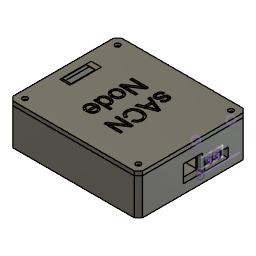
sACN Node 3xXLR_v31 (Autodesk Fusion 360 design; units mm, degrees)
Autodesk Fusion 360 part; units mm, degrees
(part 1 of 2)
sketch "Skizze1" plane through (0, 0, 0) normal (0, 1, 0) x (1, 0, 0) in component "Board"
  line L0 (99.5, 0) -> (99.5, 67)
  line L1 (99.5, 67) -> (99.5, 42.25) construction
  line L2 (99.5, 42.25) -> (99.5, 25.5) construction
  line L3 (99.5, 25.5) -> (99.5, 0) construction
  line L4 (99.5, 42.25) -> (101, 42.25)
  line L5 (101, 42.25) -> (101, 26.25)
  line L6 (101, 26.25) -> (99.5, 26.25)
  line L7 (99.5, 26.25) -> (99.5, 42.25) construction
  line L8 (99.5, 67) -> (99.5, 60.5) construction
  line L9 (99.5, 47.25) -> (99.5, 60.5)
  line L10 (99.5, -28.5) -> (0, -28.5)
  line L11 (0, 95.5) -> (99.5, 95.5)
  line L12 (99.5, 95.5) -> (99.5, -28.5)
  line L13 (0, 95.5) -> (-50, 95.5)
  line L14 (-50, 95.5) -> (-50, -28.5)
  line L15 (-50, -28.5) -> (0, -28.5)
  line L16 (0, 100.5) -> (104.5, 100.5)
  line L17 (104.5, 100.5) -> (104.5, -33.5)
  line L18 (104.5, -33.5) -> (0, -33.5)
  line L19 (-55, -33.5) -> (0, -33.5)
  line L20 (-55, 100.5) -> (-55, -33.5)
  line L21 (0, 100.5) -> (-55, 100.5)
  line L22 (99.5, 62) -> (99.5, 67)
  line L23 (99.5, 5) -> (99.5, 0)
  line L24 (99.5, 0) -> (99.5, -0.4)
  line L25 (99.5, -0.4) -> (99.5, -2.4)
  line L26 (99.5, 67.4) -> (99.5, 69.4)
  line L27 (99.5, 67) -> (99.5, 67.4)
  line L28 (99.5, 33.5) -> (99.5, 47.25)
  line L29 (99.5, 47.25) -> (41, 47.25)
  line L30 (41, 47.25) -> (41, 21.25)
  line L31 (41, 21.25) -> (99.5, 21.25)
  line L32 (99.5, 21.25) -> (99.5, 47.25)
  circle A0 centre (97.5, 45.25) radius 1
  circle A1 centre (97.5, 23.25) radius 1
  line L33 (5.6871, 39.4777, 4.3933) -> (5.6871, 41.4777, 4.3933)
  line L34 (5.6871, 39.4777, 4.3947) -> (5.6871, 41.4777, 4.3947)
  line L35 (-22.2425, 41.4777, 4.3947) -> (-22.2425, 45.4777, 4.3947) construction
  line L36 (-6.3129, 41.4777, 4.3947) -> (-6.3129, 39.4777, 4.3947)
  line L37 (-0.3129, 46.5108, 4.3947) -> (-0.3129, 40.4777, 4.3947) construction
  line L38 (-21.0987, 63.9777, 4.3931) -> (-21.0987, 41.4777, 4.3931) construction
  line L39 (-0.3129, 46.5108, 4.3932) -> (-0.3129, 40.4777, 4.3933) construction
  line L40 (-18.5761, 41.4777, 4.3947) -> (-18.5761, 33.4777, 4.3947) construction
  line L41 (5.6871, 45.5113, 4.3947) -> (5.6871, 47.5113, 4.3947)
  line L42 (16.2858, 41.4777, 4.3931) -> (16.2858, 63.9777, 4.3931) construction
  line L43 (-11.4093, 33.4777, 4.3934) -> (-11.4093, 41.4777, 4.3932) construction
  line L44 (5.6871, 45.5103, 4.3934) -> (5.6871, 47.5122, 4.393)
  line L45 (-6.3129, 47.5113, 4.3947) -> (-6.3129, 45.5113, 4.3947)
  line L46 (-6.3129, 41.4777, 4.3933) -> (-6.3129, 39.4777, 4.3933)
  line L47 (-18.5761, 33.4777, 4.3934) -> (-11.4093, 33.4777, 4.3934) construction
  line L48 (-6.3129, 47.5122, 4.393) -> (5.6871, 45.5103, 4.3934) construction
  line L49 (5.6871, 41.4777, 4.3933) -> (-6.3129, 41.4777, 4.3933)
  line L50 (5.6871, 47.5122, 4.393) -> (-6.3129, 45.5103, 4.3934) construction
  line L51 (21.2575, 45.4777, 4.3934) -> (-22.2425, 41.4777, 4.3931) construction
  line L52 (-18.5761, 41.4777, 4.3932) -> (-18.5761, 33.4777, 4.3934) construction
  line L53 (-6.3129, 39.4777, 4.3933) -> (5.6871, 39.4777, 4.3933)
  line L54 (-21.0987, 41.4777, 4.3931) -> (16.2858, 41.4777, 4.3931) construction
  line L55 (5.6871, 47.5113, 4.3947) -> (-6.3129, 47.5113, 4.3947)
  line L56 (-18.5761, 33.4777, 4.3947) -> (-11.4093, 33.4777, 4.3947) construction
  line L57 (-11.4093, 33.4777, 4.3947) -> (-11.4093, 41.4777, 4.3947) construction
  line L58 (-22.2425, 45.4777, 4.3947) -> (21.2575, 45.4777, 4.3947) construction
  line L59 (21.2575, 45.4777, 4.3947) -> (-22.2425, 41.4777, 4.3947) construction
  line L60 (-6.3129, 47.5122, 4.393) -> (-6.3129, 45.5103, 4.3934)
  line L61 (-6.3129, 47.5113, 4.3947) -> (5.6871, 45.5113, 4.3947) construction
  line L62 (-22.2425, 41.4777, 4.3931) -> (-22.2425, 45.4777, 4.3931) construction
  line L63 (21.2575, 45.4777, 4.3947) -> (21.2575, 41.4777, 4.3947) construction
  line L64 (21.2575, 45.4777, 4.3934) -> (21.2575, 41.4777, 4.3934) construction
  line L65 (5.6871, 47.5113, 4.3947) -> (-6.3129, 45.5113, 4.3947) construction
  line L66 (-22.2425, 45.4777, 4.3931) -> (21.2575, 41.4777, 4.3934) construction
  line L67 (-6.3129, 45.5113, 4.3947) -> (5.6871, 45.5113, 4.3947)
  line L68 (21.2575, 41.4777, 4.3947) -> (-22.2425, 41.4777, 4.3947) construction
  line L69 (-6.3129, 41.4777, 4.3933) -> (5.6871, 39.4777, 4.3933) construction
  line L70 (16.2858, 63.9777, 4.3931) -> (-21.0987, 63.9777, 4.3931) construction
  line L71 (5.6871, 47.5122, 4.393) -> (-6.3129, 47.5122, 4.393)
  line L72 (5.6871, 41.4777, 4.3947) -> (-6.3129, 41.4777, 4.3947)
  line L73 (-22.2425, 45.4777, 4.3947) -> (21.2575, 41.4777, 4.3947) construction
  line L74 (-6.3129, 45.5103, 4.3934) -> (5.6871, 45.5103, 4.3934)
  line L75 (-6.3129, 41.4777, 4.3947) -> (5.6871, 39.4777, 4.3947) construction
  line L76 (21.2575, 41.4777, 4.3934) -> (-22.2425, 41.4777, 4.3931) construction
  line L77 (-22.2425, 45.4777, 4.3931) -> (21.2575, 45.4777, 4.3934) construction
  line L78 (-6.3129, 39.4777, 4.3947) -> (5.6871, 39.4777, 4.3947)
  line L79 (5.6871, 41.4777, 4.3933) -> (-6.3129, 39.4777, 4.3933) construction
  line L80 (5.6871, 41.4777, 4.3947) -> (-6.3129, 39.4777, 4.3947) construction
  line L81 (-6.3129, 47.5113, 4.3932) -> (-6.3129, 45.5113, 4.3932)
  line L82 (5.6871, 39.4777, 4.3933) -> (5.6871, 41.4777, 4.3933)
  line L83 (5.6871, 41.4777, 4.3947) -> (-6.3129, 39.4777, 4.3947) construction
  line L84 (-22.2425, 45.4777, 4.3931) -> (21.2575, 45.4777, 4.3934) construction
  line L85 (-22.2425, 45.4777, 4.3947) -> (21.2575, 41.4777, 4.3947) construction
  line L86 (-18.5761, 41.4777, 4.3947) -> (-18.5761, 33.4777, 4.3947) construction
  line L87 (-22.2425, 45.4777, 4.3947) -> (21.2575, 45.4777, 4.3947) construction
  line L88 (5.6871, 47.5113, 4.3947) -> (-6.3129, 47.5113, 4.3947)
  line L89 (5.6871, 45.5113, 4.3932) -> (5.6871, 47.5113, 4.3932)
  line L90 (-6.3129, 41.4777, 4.3933) -> (5.6871, 39.4777, 4.3933) construction
  line L91 (5.6871, 45.5113, 4.3947) -> (5.6871, 47.5113, 4.3947)
  line L92 (-6.3129, 47.5113, 4.3947) -> (5.6871, 45.5113, 4.3947) construction
  line L93 (-6.3129, 41.4777, 4.3947) -> (5.6871, 39.4777, 4.3947) construction
  line L94 (5.6871, 41.4777, 4.3933) -> (-6.3129, 41.4777, 4.3933)
  line L95 (21.2575, 45.4777, 4.3934) -> (21.2575, 41.4777, 4.3934) construction
  line L96 (-0.3129, 46.5108, 4.3947) -> (-0.3129, 40.4777, 4.3947) construction
  line L97 (5.6871, 41.4777, 4.3933) -> (-6.3129, 39.4777, 4.3933) construction
  line L98 (-6.3129, 41.4777, 4.3933) -> (-6.3129, 39.4777, 4.3933)
  line L99 (5.6871, 41.4777, 4.3947) -> (-6.3129, 41.4777, 4.3947)
  line L100 (-6.3129, 39.4777, 4.3933) -> (5.6871, 39.4777, 4.3933)
  line L101 (5.6871, 47.5113, 4.3932) -> (-6.3129, 45.5113, 4.3932) construction
  line L102 (-6.3129, 45.5113, 4.3932) -> (5.6871, 45.5113, 4.3932)
  line L103 (-6.3129, 39.4777, 4.3947) -> (5.6871, 39.4777, 4.3947)
  line L104 (21.2575, 45.4777, 4.3947) -> (21.2575, 41.4777, 4.3947) construction
  line L105 (-6.3129, 47.5113, 4.3947) -> (-6.3129, 45.5113, 4.3947)
  line L106 (16.2858, 63.9777, 4.3931) -> (-21.0987, 63.9777, 4.3931) construction
  line L107 (-22.2425, 41.4777, 4.3947) -> (-22.2425, 45.4777, 4.3947) construction
  line L108 (21.2575, 41.4777, 4.3947) -> (-22.2425, 41.4777, 4.3947) construction
  line L109 (21.2575, 41.4777, 4.3934) -> (-22.2425, 41.4777, 4.3931) construction
  line L110 (-21.0987, 63.9777, 4.3931) -> (-21.0987, 41.4777, 4.3931) construction
  line L111 (-21.0987, 41.4777, 4.3931) -> (16.2858, 41.4777, 4.3931) construction
  line L112 (16.2858, 41.4777, 4.3931) -> (16.2858, 63.9777, 4.3931) construction
  line L113 (21.2575, 45.4777, 4.3947) -> (-22.2425, 41.4777, 4.3947) construction
  line L114 (-18.5761, 33.4777, 4.3947) -> (-11.4093, 33.4777, 4.3947) construction
  line L115 (-22.2425, 45.4777, 4.3931) -> (21.2575, 41.4777, 4.3934) construction
  line L116 (-18.5761, 41.4777, 4.3932) -> (-18.5761, 33.4777, 4.3934) construction
  line L117 (21.2575, 45.4777, 4.3934) -> (-22.2425, 41.4777, 4.3931) construction
  line L118 (-18.5761, 33.4777, 4.3934) -> (-11.4093, 33.4777, 4.3934) construction
  line L119 (-22.2425, 41.4777, 4.3931) -> (-22.2425, 45.4777, 4.3931) construction
  line L120 (5.6871, 39.4777, 4.3947) -> (5.6871, 41.4777, 4.3947)
  line L121 (-11.4093, 33.4777, 4.3934) -> (-11.4093, 41.4777, 4.3932) construction
  line L122 (5.6871, 47.5113, 4.3932) -> (-6.3129, 47.5113, 4.3932)
  line L123 (-11.4093, 33.4777, 4.3947) -> (-11.4093, 41.4777, 4.3947) construction
  line L124 (-6.3129, 47.5113, 4.3932) -> (5.6871, 45.5113, 4.3932) construction
  line L125 (-6.3129, 41.4777, 4.3947) -> (-6.3129, 39.4777, 4.3947)
  line L126 (-6.3129, 45.5113, 4.3947) -> (5.6871, 45.5113, 4.3947)
  line L127 (5.6871, 47.5113, 4.3947) -> (-6.3129, 45.5113, 4.3947) construction
  line L128 (-0.3129, 46.5108, 4.3932) -> (-0.3129, 40.4777, 4.3933) construction
  line L129 (21.2575, 14.9777, 4.3947) -> (21.2575, 10.9777, 4.3947) construction
  line L130 (-0.3129, 16.0108, 4.3947) -> (-0.3129, 9.9777, 4.3947) construction
  line L131 (-18.5761, 2.9777, 4.3934) -> (-11.4093, 2.9777, 4.3934) construction
  line L132 (-22.2425, 10.9777, 4.3931) -> (-22.2425, 14.9777, 4.3931) construction
  line L133 (-22.2425, 10.9777, 4.3931) -> (-22.2425, 14.9777, 4.3931) construction
  line L134 (21.2575, 14.9777, 4.3947) -> (21.2575, 10.9777, 4.3947) construction
  line L135 (-11.4093, 2.9777, 4.3947) -> (-11.4093, 10.9777, 4.3947) construction
  line L136 (-22.2425, 10.9777, 4.3947) -> (-22.2425, 14.9777, 4.3947) construction
  line L137 (21.2575, 14.9777, 4.3934) -> (21.2575, 10.9777, 4.3934) construction
  line L138 (-0.3129, 16.0108, 4.3932) -> (-0.3129, 9.9777, 4.3933) construction
  line L139 (-0.3129, 16.0108, 4.3947) -> (-0.3129, 9.9777, 4.3947) construction
  line L140 (21.2575, 14.9777, 4.3934) -> (21.2575, 10.9777, 4.3934) construction
  line L141 (-18.5761, 10.9777, 4.3932) -> (-18.5761, 2.9777, 4.3934) construction
  line L142 (21.2575, 14.9777, 4.3934) -> (-22.2425, 10.9777, 4.3931) construction
  line L143 (-22.2425, 14.9777, 4.3931) -> (21.2575, 14.9777, 4.3934) construction
  line L144 (21.2575, 10.9777, 4.3934) -> (-22.2425, 10.9777, 4.3931) construction
  line L145 (-22.2425, 14.9777, 4.3931) -> (21.2575, 10.9777, 4.3934) construction
  line L146 (21.2575, 14.9777, 4.3934) -> (-22.2425, 10.9777, 4.3931) construction
  line L147 (-0.3129, 16.0108, 4.3932) -> (-0.3129, 9.9777, 4.3933) construction
  line L148 (-18.5761, 2.9777, 4.3947) -> (-11.4093, 2.9777, 4.3947) construction
  line L149 (-11.4093, 2.9777, 4.3947) -> (-11.4093, 10.9777, 4.3947) construction
  line L150 (-11.4093, 2.9777, 4.3934) -> (-11.4093, 10.9777, 4.3932) construction
  line L151 (-11.4093, 2.9777, 4.3934) -> (-11.4093, 10.9777, 4.3932) construction
  line L152 (-22.2425, 10.9777, 4.3947) -> (-22.2425, 14.9777, 4.3947) construction
  line L153 (-6.3129, 17.0113, 4.3947) -> (-6.3129, 15.0113, 4.3947)
  line L154 (-6.3129, 10.9777, 4.3933) -> (5.6871, 8.9777, 4.3933) construction
  line L155 (-18.5761, 2.9777, 4.3947) -> (-11.4093, 2.9777, 4.3947) construction
  line L156 (5.6871, 15.0113, 4.3947) -> (5.6871, 17.0113, 4.3947)
  line L157 (5.6871, 17.0113, 4.3947) -> (-6.3129, 17.0113, 4.3947)
  line L158 (-18.5761, 10.9777, 4.3947) -> (-18.5761, 2.9777, 4.3947) construction
  line L159 (5.6871, 17.0113, 4.3932) -> (-6.3129, 15.0113, 4.3932) construction
  line L160 (5.6871, 10.9777, 4.3947) -> (-6.3129, 8.9777, 4.3947) construction
  line L161 (-18.5761, 2.9777, 4.3934) -> (-11.4093, 2.9777, 4.3934) construction
  line L162 (-6.3129, 15.0113, 4.3932) -> (5.6871, 15.0113, 4.3932)
  line L163 (-6.3129, 10.9777, 4.3933) -> (5.6871, 8.9777, 4.3933) construction
  line L164 (5.6871, 17.0113, 4.3932) -> (-6.3129, 15.0113, 4.3932) construction
  line L165 (-6.3129, 8.9777, 4.3933) -> (5.6871, 8.9777, 4.3933)
  line L166 (5.6871, 8.9777, 4.3947) -> (5.6871, 10.9777, 4.3947)
  line L167 (5.6871, 17.0113, 4.3932) -> (-6.3129, 17.0113, 4.3932)
  line L168 (-6.3129, 10.9777, 4.3947) -> (5.6871, 8.9777, 4.3947) construction
  line L169 (5.6871, 15.0113, 4.3932) -> (5.6871, 17.0113, 4.3932)
  line L170 (-18.5761, 10.9777, 4.3932) -> (-18.5761, 2.9777, 4.3934) construction
  line L171 (-6.3129, 15.0113, 4.3947) -> (5.6871, 15.0113, 4.3947)
  line L172 (5.6871, 10.9777, 4.3933) -> (-6.3129, 8.9777, 4.3933) construction
  line L173 (5.6871, 8.9777, 4.3933) -> (5.6871, 10.9777, 4.3933)
  line L174 (-6.3129, 17.0113, 4.3947) -> (5.6871, 15.0113, 4.3947) construction
  line L175 (-6.3129, 10.9777, 4.3947) -> (-6.3129, 8.9777, 4.3947)
  line L176 (5.6871, 17.0113, 4.3947) -> (-6.3129, 15.0113, 4.3947) construction
  line L177 (-6.3129, 17.0113, 4.3932) -> (-6.3129, 15.0113, 4.3932)
  line L178 (-6.3129, 17.0113, 4.3932) -> (5.6871, 15.0113, 4.3932) construction
  line L179 (5.6871, 8.9777, 4.3933) -> (5.6871, 10.9777, 4.3933)
  line L180 (5.6871, 8.9777, 4.3947) -> (5.6871, 10.9777, 4.3947)
  line L181 (5.6871, 10.9777, 4.3947) -> (-6.3129, 10.9777, 4.3947)
  line L182 (5.6871, 15.0113, 4.3947) -> (5.6871, 17.0113, 4.3947)
  line L183 (-6.3129, 10.9777, 4.3947) -> (5.6871, 8.9777, 4.3947) construction
  line L184 (5.6871, 15.0113, 4.3932) -> (5.6871, 17.0113, 4.3932)
  line L185 (-6.3129, 17.0113, 4.3947) -> (-6.3129, 15.0113, 4.3947)
  line L186 (5.6871, 17.0113, 4.3932) -> (-6.3129, 17.0113, 4.3932)
  line L187 (-6.3129, 8.9777, 4.3947) -> (5.6871, 8.9777, 4.3947)
  line L188 (5.6871, 17.0113, 4.3947) -> (-6.3129, 15.0113, 4.3947) construction
  line L189 (-6.3129, 17.0113, 4.3947) -> (5.6871, 15.0113, 4.3947) construction
  line L190 (-6.3129, 17.0113, 4.3932) -> (-6.3129, 15.0113, 4.3932)
  line L191 (-6.3129, 15.0113, 4.3932) -> (5.6871, 15.0113, 4.3932)
  line L192 (-6.3129, 17.0113, 4.3932) -> (5.6871, 15.0113, 4.3932) construction
  line L193 (-6.3129, 15.0113, 4.3947) -> (5.6871, 15.0113, 4.3947)
  line L194 (5.6871, 10.9777, 4.3933) -> (-6.3129, 10.9777, 4.3933)
  line L195 (5.6871, 10.9777, 4.3947) -> (-6.3129, 10.9777, 4.3947)
  line L196 (-6.3129, 10.9777, 4.3933) -> (-6.3129, 8.9777, 4.3933)
  line L197 (5.6871, 17.0113, 4.3947) -> (-6.3129, 17.0113, 4.3947)
  line L198 (-6.3129, 8.9777, 4.3947) -> (5.6871, 8.9777, 4.3947)
  line L199 (-6.3129, 10.9777, 4.3947) -> (-6.3129, 8.9777, 4.3947)
  line L200 (5.6871, 10.9777, 4.3933) -> (-6.3129, 10.9777, 4.3933)
  line L201 (-6.3129, 10.9777, 4.3933) -> (-6.3129, 8.9777, 4.3933)
  line L202 (5.6871, 10.9777, 4.3933) -> (-6.3129, 8.9777, 4.3933) construction
  line L203 (5.6871, 10.9777, 4.3947) -> (-6.3129, 8.9777, 4.3947) construction
  line L204 (-6.3129, 8.9777, 4.3933) -> (5.6871, 8.9777, 4.3933)
  line L205 (-22.2425, 14.9777, 4.3947) -> (21.2575, 14.9777, 4.3947) construction
  line L206 (21.2575, 14.9777, 4.3947) -> (-22.2425, 10.9777, 4.3947) construction
  line L207 (-22.2425, 14.9777, 4.3947) -> (21.2575, 10.9777, 4.3947) construction
  line L208 (-18.5761, 10.9777, 4.3947) -> (-18.5761, 2.9777, 4.3947) construction
  line L209 (21.2575, 10.9777, 4.3947) -> (-22.2425, 10.9777, 4.3947) construction
  line L210 (-21.0987, 10.9777, 4.3931) -> (16.2858, 10.9777, 4.3931) construction
  line L211 (21.2575, 10.9777, 4.3934) -> (-22.2425, 10.9777, 4.3931) construction
  line L212 (-21.0987, 10.9777, 4.3931) -> (16.2858, 10.9777, 4.3931) construction
  line L213 (-22.2425, 14.9777, 4.3931) -> (21.2575, 10.9777, 4.3934) construction
  line L214 (-22.2425, 14.9777, 4.3931) -> (21.2575, 14.9777, 4.3934) construction
  line L215 (16.2858, 10.9777, 4.3931) -> (16.2858, 33.4777, 4.3931) construction
  line L216 (-21.0987, 33.4777, 4.3931) -> (-21.0987, 10.9777, 4.3931) construction
  line L217 (21.2575, 14.9777, 4.3947) -> (-22.2425, 10.9777, 4.3947) construction
  line L218 (-21.0987, 33.4777, 4.3931) -> (-21.0987, 10.9777, 4.3931) construction
  line L219 (16.2858, 33.4777, 4.3931) -> (-21.0987, 33.4777, 4.3931) construction
  line L220 (16.2858, 33.4777, 4.3931) -> (-21.0987, 33.4777, 4.3931) construction
  line L221 (-22.2425, 14.9777, 4.3947) -> (21.2575, 14.9777, 4.3947) construction
  line L222 (21.2575, 10.9777, 4.3947) -> (-22.2425, 10.9777, 4.3947) construction
  line L223 (-22.2425, 14.9777, 4.3947) -> (21.2575, 10.9777, 4.3947) construction
  line L224 (16.2858, 10.9777, 4.3931) -> (16.2858, 33.4777, 4.3931) construction
  line L225 (21.2575, 75.9777, 4.3946) -> (21.2575, 71.9777, 4.3946) construction
  line L226 (-0.3132, 77.0107, 4.3946) -> (-0.3132, 70.9777, 4.3946) construction
  line L227 (-18.5761, 63.9777, 4.3934) -> (-11.4093, 63.9777, 4.3934) construction
  line L228 (-22.2425, 71.9777, 4.3931) -> (-22.2425, 75.9777, 4.3931) construction
  line L229 (-22.2425, 71.9777, 4.3931) -> (-22.2425, 75.9777, 4.3931) construction
  line L230 (21.2575, 75.9777, 4.3947) -> (21.2575, 71.9777, 4.3947) construction
  line L231 (-11.4093, 63.9777, 4.3946) -> (-11.4093, 71.9777, 4.3946) construction
  line L232 (-22.2425, 71.9777, 4.3947) -> (-22.2425, 75.9777, 4.3947) construction
  line L233 (21.2575, 75.9777, 4.3934) -> (21.2575, 71.9777, 4.3934) construction
  line L234 (-0.3129, 77.0108, 4.3932) -> (-0.3129, 70.9777, 4.3933) construction
  line L235 (-0.3129, 77.0108, 4.3947) -> (-0.3129, 70.9777, 4.3947) construction
  line L236 (21.2575, 75.9777, 4.3934) -> (21.2575, 71.9777, 4.3934) construction
  line L237 (-18.5761, 71.9777, 4.3932) -> (-18.5761, 63.9777, 4.3934) construction
  line L238 (21.2575, 75.9777, 4.3934) -> (-22.2425, 71.9777, 4.3931) construction
  line L239 (-22.2425, 75.9777, 4.3931) -> (21.2575, 75.9777, 4.3934) construction
  line L240 (21.2575, 71.9777, 4.3934) -> (-22.2425, 71.9777, 4.3931) construction
  line L241 (-22.2425, 75.9777, 4.3931) -> (21.2575, 71.9777, 4.3934) construction
  line L242 (21.2575, 75.9777, 4.3934) -> (-22.2425, 71.9777, 4.3931) construction
  line L243 (-0.3129, 77.0108, 4.3932) -> (-0.3129, 70.9777, 4.3933) construction
  line L244 (-18.5761, 63.9777, 4.3946) -> (-11.4093, 63.9777, 4.3946) construction
  line L245 (-11.4093, 63.9777, 4.3947) -> (-11.4093, 71.9777, 4.3947) construction
  line L246 (-11.4093, 63.9777, 4.3934) -> (-11.4093, 71.9777, 4.3932) construction
  line L247 (-11.4093, 63.9777, 4.3934) -> (-11.4093, 71.9777, 4.3932) construction
  line L248 (-22.2425, 71.9777, 4.3946) -> (-22.2425, 75.9777, 4.3946) construction
  line L249 (-6.3132, 78.0113, 4.3946) -> (-6.3132, 76.0113, 4.3946)
  line L250 (-6.3129, 71.9777, 4.3933) -> (5.6871, 71.9777, 4.3933)
  line L251 (-6.3129, 71.9777, 4.3933) -> (5.6871, 69.9777, 4.3933) construction
  line L252 (-18.5761, 63.9777, 4.3947) -> (-11.4093, 63.9777, 4.3947) construction
  line L253 (5.6868, 76.0113, 4.3946) -> (5.6868, 78.0113, 4.3946)
  line L254 (5.6871, 78.0113, 4.3947) -> (-6.3129, 78.0113, 4.3947)
  line L255 (-18.5761, 71.9777, 4.3946) -> (-18.5761, 63.9777, 4.3946) construction
  line L256 (5.6871, 78.0113, 4.3932) -> (-6.3129, 76.0113, 4.3932) construction
  line L257 (-6.3129, 71.9777, 4.3933) -> (5.6871, 71.9777, 4.3933)
  line L258 (5.6868, 71.9777, 4.3946) -> (-6.3132, 69.9777, 4.3946) construction
  line L259 (-18.5761, 63.9777, 4.3934) -> (-11.4093, 63.9777, 4.3934) construction
  line L260 (-6.3129, 76.0113, 4.3932) -> (5.6871, 76.0113, 4.3932)
  line L261 (-6.3129, 71.9777, 4.3933) -> (5.6871, 69.9777, 4.3933) construction
  line L262 (5.6871, 78.0113, 4.3932) -> (-6.3129, 76.0113, 4.3932) construction
  line L263 (-6.3129, 69.9777, 4.3933) -> (5.6871, 69.9777, 4.3933)
  line L264 (5.6871, 69.9777, 4.3947) -> (5.6871, 71.9777, 4.3947)
  line L265 (5.6871, 78.0113, 4.3932) -> (-6.3129, 78.0113, 4.3932)
  line L266 (-6.3129, 71.9777, 4.3947) -> (5.6871, 69.9777, 4.3947) construction
  line L267 (5.6871, 76.0113, 4.3932) -> (5.6871, 78.0113, 4.3932)
  line L268 (-18.5761, 71.9777, 4.3932) -> (-18.5761, 63.9777, 4.3934) construction
  line L269 (-6.3129, 76.0113, 4.3947) -> (5.6871, 76.0113, 4.3947)
  line L270 (5.6871, 71.9777, 4.3933) -> (-6.3129, 69.9777, 4.3933) construction
  line L271 (5.6871, 69.9777, 4.3933) -> (5.6871, 71.9777, 4.3933)
  line L272 (-6.3132, 78.0113, 4.3946) -> (5.6868, 76.0113, 4.3946) construction
  line L273 (-6.3129, 71.9777, 4.3947) -> (-6.3129, 69.9777, 4.3947)
  line L274 (5.6868, 78.0113, 4.3946) -> (-6.3132, 76.0113, 4.3946) construction
  line L275 (-6.3129, 78.0113, 4.3932) -> (-6.3129, 76.0113, 4.3932)
  line L276 (-6.3129, 78.0113, 4.3932) -> (5.6871, 76.0113, 4.3932) construction
  line L277 (5.6871, 69.9777, 4.3933) -> (5.6871, 71.9777, 4.3933)
  line L278 (5.6868, 69.9777, 4.3946) -> (5.6868, 71.9777, 4.3946)
  line L279 (5.6868, 71.9777, 4.3946) -> (-6.3132, 71.9777, 4.3946)
  line L280 (5.6871, 76.0113, 4.3947) -> (5.6871, 78.0113, 4.3947)
  line L281 (-6.3129, 71.9777, 4.3933) -> (5.6871, 71.9777, 4.3933)
  line L282 (-6.3132, 71.9777, 4.3946) -> (5.6868, 69.9777, 4.3946) construction
  line L283 (5.6871, 76.0113, 4.3932) -> (5.6871, 78.0113, 4.3932)
  line L284 (-6.3129, 78.0113, 4.3947) -> (-6.3129, 76.0113, 4.3947)
  line L285 (5.6871, 78.0113, 4.3932) -> (-6.3129, 78.0113, 4.3932)
  line L286 (-6.3132, 69.9777, 4.3946) -> (5.6868, 69.9777, 4.3946)
  line L287 (5.6871, 78.0113, 4.3947) -> (-6.3129, 76.0113, 4.3947) construction
  line L288 (-6.3129, 78.0113, 4.3947) -> (5.6871, 76.0113, 4.3947) construction
  line L289 (-6.3129, 71.9777, 4.3933) -> (5.6871, 71.9777, 4.3933)
  line L290 (-6.3129, 78.0113, 4.3932) -> (-6.3129, 76.0113, 4.3932)
  line L291 (-6.3129, 76.0113, 4.3932) -> (5.6871, 76.0113, 4.3932)
  line L292 (-6.3129, 78.0113, 4.3932) -> (5.6871, 76.0113, 4.3932) construction
  line L293 (-6.3132, 76.0113, 4.3946) -> (5.6868, 76.0113, 4.3946)
  line L294 (5.6871, 71.9777, 4.3933) -> (-6.3129, 71.9777, 4.3933)
  line L295 (5.6871, 71.9777, 4.3947) -> (-6.3129, 71.9777, 4.3947)
  line L296 (-6.3129, 71.9777, 4.3933) -> (-6.3129, 69.9777, 4.3933)
  line L297 (5.6868, 78.0113, 4.3946) -> (-6.3132, 78.0113, 4.3946)
  line L298 (-6.3129, 69.9777, 4.3947) -> (5.6871, 69.9777, 4.3947)
  line L299 (-6.3132, 71.9777, 4.3946) -> (-6.3132, 69.9777, 4.3946)
  line L300 (5.6871, 71.9777, 4.3933) -> (-6.3129, 71.9777, 4.3933)
  line L301 (-6.3129, 71.9777, 4.3933) -> (-6.3129, 69.9777, 4.3933)
  line L302 (5.6871, 71.9777, 4.3933) -> (-6.3129, 69.9777, 4.3933) construction
  line L303 (5.6871, 71.9777, 4.3947) -> (-6.3129, 69.9777, 4.3947) construction
  line L304 (-6.3129, 69.9777, 4.3933) -> (5.6871, 69.9777, 4.3933)
  line L305 (-22.2425, 75.9777, 4.3946) -> (21.2575, 75.9777, 4.3946) construction
  line L306 (21.2575, 75.9777, 4.3946) -> (-22.2425, 71.9777, 4.3946) construction
  line L307 (-22.2425, 75.9777, 4.3947) -> (21.2575, 71.9777, 4.3947) construction
  line L308 (-18.5761, 71.9777, 4.3947) -> (-18.5761, 63.9777, 4.3947) construction
  line L309 (21.2575, 71.9777, 4.3946) -> (-22.2425, 71.9777, 4.3946) construction
  line L310 (-21.0987, 71.9777, 4.3931) -> (16.2858, 71.9777, 4.3931) construction
  line L311 (21.2575, 71.9777, 4.3934) -> (-22.2425, 71.9777, 4.3931) construction
  line L312 (-21.0987, 71.9777, 4.3931) -> (16.2858, 71.9777, 4.3931) construction
  line L313 (-22.2425, 75.9777, 4.3931) -> (21.2575, 71.9777, 4.3934) construction
  line L314 (-22.2425, 75.9777, 4.3931) -> (21.2575, 75.9777, 4.3934) construction
  line L315 (16.2858, 71.9777, 4.3931) -> (16.2858, 94.4777, 4.3931) construction
  line L316 (-21.0987, 94.4777, 4.3931) -> (-21.0987, 71.9777, 4.3931) construction
  line L317 (21.2575, 75.9777, 4.3947) -> (-22.2425, 71.9777, 4.3947) construction
  line L318 (-21.0987, 94.4777, 4.3931) -> (-21.0987, 71.9777, 4.3931) construction
  line L319 (16.2858, 94.4777, 4.3931) -> (-21.0987, 94.4777, 4.3931) construction
  line L320 (16.2858, 94.4777, 4.3931) -> (-21.0987, 94.4777, 4.3931) construction
  line L321 (-22.2425, 75.9777, 4.3947) -> (21.2575, 75.9777, 4.3947) construction
  line L322 (21.2575, 71.9777, 4.3947) -> (-22.2425, 71.9777, 4.3947) construction
  line L323 (-22.2425, 75.9777, 4.3946) -> (21.2575, 71.9777, 4.3946) construction
  line L324 (16.2858, 71.9777, 4.3931) -> (16.2858, 94.4777, 4.3931) construction
  line L325 (21.2575, -15.5223, 4.3947) -> (21.2575, -19.5223, 4.3947) construction
  line L326 (-0.3129, -14.4892, 4.3947) -> (-0.3129, -20.5223, 4.3947) construction
  line L327 (-18.5761, -27.5223, 4.3934) -> (-11.4093, -27.5223, 4.3934) construction
  line L328 (-22.2425, -19.5223, 4.3931) -> (-22.2425, -15.5223, 4.3931) construction
  line L329 (-22.2425, -19.5223, 4.3931) -> (-22.2425, -15.5223, 4.3931) construction
  line L330 (21.2575, -15.5223, 4.3947) -> (21.2575, -19.5223, 4.3947) construction
  line L331 (-11.4093, -27.5223, 4.3947) -> (-11.4093, -19.5223, 4.3947) construction
  line L332 (-22.2425, -19.5223, 4.3947) -> (-22.2425, -15.5223, 4.3947) construction
  line L333 (21.2575, -15.5223, 4.3934) -> (21.2575, -19.5223, 4.3934) construction
  line L334 (-0.3129, -14.4892, 4.3932) -> (-0.3129, -20.5223, 4.3933) construction
  line L335 (-0.3129, -14.4892, 4.3947) -> (-0.3129, -20.5223, 4.3947) construction
  line L336 (21.2575, -15.5223, 4.3934) -> (21.2575, -19.5223, 4.3934) construction
  line L337 (-18.5761, -19.5223, 4.3932) -> (-18.5761, -27.5223, 4.3934) construction
  line L338 (21.2575, -15.5223, 4.3934) -> (-22.2425, -19.5223, 4.3931) construction
  line L339 (-22.2425, -15.5223, 4.3931) -> (21.2575, -15.5223, 4.3934) construction
  line L340 (21.2575, -19.5223, 4.3934) -> (-22.2425, -19.5223, 4.3931) construction
  line L341 (-22.2425, -15.5223, 4.3931) -> (21.2575, -19.5223, 4.3934) construction
  line L342 (21.2575, -15.5223, 4.3934) -> (-22.2425, -19.5223, 4.3931) construction
  line L343 (-0.3129, -14.4892, 4.3932) -> (-0.3129, -20.5223, 4.3933) construction
  line L344 (-18.5761, -27.5223, 4.3947) -> (-11.4093, -27.5223, 4.3947) construction
  line L345 (-11.4093, -27.5223, 4.3947) -> (-11.4093, -19.5223, 4.3947) construction
  line L346 (-11.4093, -27.5223, 4.3934) -> (-11.4093, -19.5223, 4.3932) construction
  line L347 (-11.4093, -27.5223, 4.3934) -> (-11.4093, -19.5223, 4.3932) construction
  line L348 (-22.2425, -19.5223, 4.3947) -> (-22.2425, -15.5223, 4.3947) construction
  line L349 (-6.3129, -13.4887, 4.3947) -> (-6.3129, -15.4887, 4.3947)
  line L350 (-6.3129, -19.5223, 4.3933) -> (5.6871, -19.5223, 4.3933)
  line L351 (-6.3129, -19.5223, 4.3933) -> (5.6871, -21.5223, 4.3933) construction
  line L352 (-18.5761, -27.5223, 4.3947) -> (-11.4093, -27.5223, 4.3947) construction
  line L353 (5.6871, -15.4887, 4.3947) -> (5.6871, -13.4887, 4.3947)
  line L354 (5.6871, -13.4887, 4.3947) -> (-6.3129, -13.4887, 4.3947)
  line L355 (-18.5761, -19.5223, 4.3947) -> (-18.5761, -27.5223, 4.3947) construction
  line L356 (5.6871, -13.4887, 4.3932) -> (-6.3129, -15.4887, 4.3932) construction
  line L357 (-6.3129, -19.5223, 4.3933) -> (5.6871, -19.5223, 4.3933)
  line L358 (5.6871, -19.5223, 4.3947) -> (-6.3129, -21.5223, 4.3947) construction
  line L359 (-18.5761, -27.5223, 4.3934) -> (-11.4093, -27.5223, 4.3934) construction
  line L360 (-6.3129, -15.4887, 4.3932) -> (5.6871, -15.4887, 4.3932)
  line L361 (-6.3129, -19.5223, 4.3933) -> (5.6871, -21.5223, 4.3933) construction
  line L362 (5.6871, -13.4887, 4.3932) -> (-6.3129, -15.4887, 4.3932) construction
  line L363 (-6.3129, -21.5223, 4.3933) -> (5.6871, -21.5223, 4.3933)
  line L364 (5.6871, -21.5223, 4.3947) -> (5.6871, -19.5223, 4.3947)
  line L365 (5.6871, -13.4887, 4.3932) -> (-6.3129, -13.4887, 4.3932)
  line L366 (-6.3129, -19.5223, 4.3947) -> (5.6871, -21.5223, 4.3947) construction
  line L367 (5.6871, -15.4887, 4.3932) -> (5.6871, -13.4887, 4.3932)
  line L368 (-18.5761, -19.5223, 4.3932) -> (-18.5761, -27.5223, 4.3934) construction
  line L369 (-6.3129, -15.4887, 4.3947) -> (5.6871, -15.4887, 4.3947)
  line L370 (5.6871, -19.5223, 4.3933) -> (-6.3129, -21.5223, 4.3933) construction
  line L371 (5.6871, -21.5223, 4.3933) -> (5.6871, -19.5223, 4.3933)
  line L372 (-6.3129, -13.4887, 4.3947) -> (5.6871, -15.4887, 4.3947) construction
  line L373 (-6.3129, -19.5223, 4.3947) -> (-6.3129, -21.5223, 4.3947)
  line L374 (5.6871, -13.4887, 4.3947) -> (-6.3129, -15.4887, 4.3947) construction
  line L375 (-6.3129, -13.4887, 4.3932) -> (-6.3129, -15.4887, 4.3932)
  line L376 (-6.3129, -13.4887, 4.3932) -> (5.6871, -15.4887, 4.3932) construction
  line L377 (5.6871, -21.5223, 4.3933) -> (5.6871, -19.5223, 4.3933)
  line L378 (5.6871, -21.5223, 4.3947) -> (5.6871, -19.5223, 4.3947)
  line L379 (5.6871, -19.5223, 4.3947) -> (-6.3129, -19.5223, 4.3947)
  line L380 (5.6871, -15.4887, 4.3947) -> (5.6871, -13.4887, 4.3947)
  line L381 (-6.3129, -19.5223, 4.3933) -> (5.6871, -19.5223, 4.3933)
  line L382 (-6.3129, -19.5223, 4.3947) -> (5.6871, -21.5223, 4.3947) construction
  line L383 (5.6871, -15.4887, 4.3932) -> (5.6871, -13.4887, 4.3932)
  line L384 (-6.3129, -13.4887, 4.3947) -> (-6.3129, -15.4887, 4.3947)
  line L385 (5.6871, -13.4887, 4.3932) -> (-6.3129, -13.4887, 4.3932)
  line L386 (-6.3129, -21.5223, 4.3947) -> (5.6871, -21.5223, 4.3947)
  line L387 (5.6871, -13.4887, 4.3947) -> (-6.3129, -15.4887, 4.3947) construction
  line L388 (-6.3129, -13.4887, 4.3947) -> (5.6871, -15.4887, 4.3947) construction
  line L389 (-6.3129, -19.5223, 4.3933) -> (5.6871, -19.5223, 4.3933)
  line L390 (-6.3129, -13.4887, 4.3932) -> (-6.3129, -15.4887, 4.3932)
  line L391 (-6.3129, -15.4887, 4.3932) -> (5.6871, -15.4887, 4.3932)
  line L392 (-6.3129, -13.4887, 4.3932) -> (5.6871, -15.4887, 4.3932) construction
  line L393 (-6.3129, -15.4887, 4.3947) -> (5.6871, -15.4887, 4.3947)
  line L394 (5.6871, -19.5223, 4.3933) -> (-6.3129, -19.5223, 4.3933)
  line L395 (5.6871, -19.5223, 4.3947) -> (-6.3129, -19.5223, 4.3947)
  line L396 (-6.3129, -19.5223, 4.3933) -> (-6.3129, -21.5223, 4.3933)
  line L397 (5.6871, -13.4887, 4.3947) -> (-6.3129, -13.4887, 4.3947)
  line L398 (-6.3129, -21.5223, 4.3947) -> (5.6871, -21.5223, 4.3947)
  line L399 (-6.3129, -19.5223, 4.3947) -> (-6.3129, -21.5223, 4.3947)
  line L400 (5.6871, -19.5223, 4.3933) -> (-6.3129, -19.5223, 4.3933)
  line L401 (-6.3129, -19.5223, 4.3933) -> (-6.3129, -21.5223, 4.3933)
  line L402 (5.6871, -19.5223, 4.3933) -> (-6.3129, -21.5223, 4.3933) construction
  line L403 (5.6871, -19.5223, 4.3947) -> (-6.3129, -21.5223, 4.3947) construction
  line L404 (-6.3129, -21.5223, 4.3933) -> (5.6871, -21.5223, 4.3933)
  line L405 (-22.2425, -15.5223, 4.3947) -> (21.2575, -15.5223, 4.3947) construction
  line L406 (21.2575, -15.5223, 4.3947) -> (-22.2425, -19.5223, 4.3947) construction
  line L407 (-22.2425, -15.5223, 4.3947) -> (21.2575, -19.5223, 4.3947) construction
  line L408 (-18.5761, -19.5223, 4.3947) -> (-18.5761, -27.5223, 4.3947) construction
  line L409 (21.2575, -19.5223, 4.3947) -> (-22.2425, -19.5223, 4.3947) construction
  line L410 (-21.0987, -19.5223, 4.3931) -> (16.2858, -19.5223, 4.3931) construction
  line L411 (21.2575, -19.5223, 4.3934) -> (-22.2425, -19.5223, 4.3931) construction
  line L412 (-21.0987, -19.5223, 4.3931) -> (16.2858, -19.5223, 4.3931) construction
  line L413 (-22.2425, -15.5223, 4.3931) -> (21.2575, -19.5223, 4.3934) construction
  line L414 (-22.2425, -15.5223, 4.3931) -> (21.2575, -15.5223, 4.3934) construction
  line L415 (16.2858, -19.5223, 4.3931) -> (16.2858, 2.9777, 4.3931) construction
  line L416 (-21.0987, 2.9777, 4.3931) -> (-21.0987, -19.5223, 4.3931) construction
  line L417 (21.2575, -15.5223, 4.3947) -> (-22.2425, -19.5223, 4.3947) construction
  line L418 (-21.0987, 2.9777, 4.3931) -> (-21.0987, -19.5223, 4.3931) construction
  line L419 (16.2858, 2.9777, 4.3931) -> (-21.0987, 2.9777, 4.3931) construction
  line L420 (16.2858, 2.9777, 4.3931) -> (-21.0987, 2.9777, 4.3931) construction
  line L421 (-22.2425, -15.5223, 4.3947) -> (21.2575, -15.5223, 4.3947) construction
  line L422 (21.2575, -19.5223, 4.3947) -> (-22.2425, -19.5223, 4.3947) construction
  line L423 (-22.2425, -15.5223, 4.3947) -> (21.2575, -19.5223, 4.3947) construction
  line L424 (16.2858, -19.5223, 4.3931) -> (16.2858, 2.9777, 4.3931) construction
  point P0 (-0.3129, 43.4943)
  point P1 (-0.3129, 40.4777)
  point P2 (-0.3129, 46.5113)
  point P3 (-0.3129, 46.5113)
  point P4 (-0.3129, 43.4943)
  point P5 (-0.3129, 40.4777)
  point P6 (-0.3129, 46.5113)
  point P7 (-0.3129, 46.5113)
  point P8 (-0.3129, 46.5113)
  point P9 (-0.3129, 46.5113)
  point P10 (-0.3129, 46.5113)
  point P11 (-0.3129, 43.4943)
  point P12 (-0.3129, 40.4777)
  point P13 (-0.3129, 46.5113)
  point P14 (-0.3129, 40.4777)
  point P15 (-0.3129, 43.4943)
  point P16 (-0.3129, 16.0113)
  point P17 (-0.3129, 16.0113)
  point P18 (-0.3129, 9.9777)
  point P19 (-0.3129, 16.0113)
  point P20 (-0.3129, 12.9943)
  point P21 (-0.3129, 16.0113)
  point P22 (-0.3129, 16.0113)
  point P23 (-0.3129, 16.0113)
  point P24 (-0.3129, 16.0113)
  point P25 (-0.3129, 12.9943)
  point P26 (-0.3129, 9.9777)
  point P27 (-0.3129, 16.0113)
  point P28 (-0.3129, 9.9777)
  point P29 (-0.3129, 12.9943)
  point P30 (-0.3129, 9.9777)
  point P31 (-0.3129, 12.9943)
  point P32 (-0.3129, 77.0113)
  point P33 (-0.3129, 77.0113)
  point P34 (-0.3129, 70.9777)
  point P35 (-0.3129, 77.0113)
  point P36 (-0.3129, 73.9943)
  point P37 (-0.3129, 77.0113)
  point P38 (-0.3132, 77.0113)
  point P39 (-0.3132, 77.0113)
  point P40 (-0.3129, 77.0113)
  point P41 (-0.3129, 73.9943)
  point P42 (-0.3129, 70.9777)
  point P43 (-0.3129, 77.0113)
  point P44 (-0.3129, 70.9777)
  point P45 (-0.3129, 73.9943)
  point P46 (-0.3132, 70.9777)
  point P47 (-0.3132, 73.9942)
  point P48 (-0.3129, -14.4887)
  point P49 (-0.3129, -14.4887)
  point P50 (-0.3129, -20.5223)
  point P51 (-0.3129, -14.4887)
  point P52 (-0.3129, -17.5057)
  point P53 (-0.3129, -14.4887)
  point P54 (-0.3129, -14.4887)
  point P55 (-0.3129, -14.4887)
  point P56 (-0.3129, -14.4887)
  point P57 (-0.3129, -17.5057)
  point P58 (-0.3129, -20.5223)
  point P59 (-0.3129, -14.4887)
  point P60 (-0.3129, -20.5223)
  point P61 (-0.3129, -17.5057)
  point P62 (-0.3129, -20.5223)
  point P63 (-0.3129, -17.5057)
  dimension "d8" = 1.5
  dimension "d26" = 124
  dimension "d27" = 50
  dimension "d28" = -5
  dimension "d132" = 159.5
  dimension "d137" = 58.5
  dimension "d138" = 26
  dimension "d139" = 2
  dimension "d140" = 2
  dimension "d145" = 2
  dimension "d146" = 2
  dimension "d147" = 2
  dimension "d148" = 2
  dimension "d181" = 5
  dimension "d182" = 16
  dimension "d184" = 5
  dimension "d272" = 43.5
  dimension "d273" = 4
  dimension "d274" = 12
  dimension "d275" = 1
  dimension "d276" = 12
  dimension "d278" = 12
  dimension "d279" = 43.5
  dimension "d280" = 4
  dimension "d281" = 12
  dimension "d282" = 1
  dimension "d283" = 12
  dimension "d285" = 12
  dimension "d286" = 22.5
  dimension "d287" = 43.5
  dimension "d288" = 4
  dimension "d289" = 12
  dimension "d290" = 1
  dimension "d291" = 12
  dimension "d293" = 12
  dimension "d294" = 43.5
  dimension "d295" = 4
  dimension "d296" = 12
  dimension "d297" = 1
  dimension "d298" = 12
  dimension "d300" = 12
  dimension "d301" = 22.5
  dimension "d302" = 43.5
  dimension "d303" = 4
  dimension "d304" = 12
  dimension "d305" = 1
  dimension "d306" = 12
  dimension "d308" = 12
  dimension "d309" = 43.5
  dimension "d310" = 4
  dimension "d311" = 12
  dimension "d312" = 1
  dimension "d313" = 12
  dimension "d315" = 12
  dimension "d316" = 22.5
  dimension "d317" = 43.5
  dimension "d318" = 4
  dimension "d319" = 12
  dimension "d320" = 1
  dimension "d321" = 12
  dimension "d323" = 12
  dimension "d324" = 43.5
  dimension "d325" = 4
  dimension "d326" = 12
  dimension "d327" = 1
  dimension "d328" = 12
  dimension "d330" = 12
  dimension "d331" = 22.5
  dimension "d332" = 43.5
  dimension "d333" = 4
  dimension "d334" = 12
  dimension "d335" = 1
  dimension "d336" = 12
  dimension "d337" = 12
  dimension "d338" = 12
  dimension "d339" = 43.5
  dimension "d340" = 4
  dimension "d341" = 12
  dimension "d342" = 1
  dimension "d343" = 12
  dimension "d344" = 12
  dimension "d345" = 12
  dimension "d346" = 22.5
  dimension "d347" = 43.5
  dimension "d348" = 4
  dimension "d349" = 12
  dimension "d350" = 1
  dimension "d351" = 12
  dimension "d352" = 12
  dimension "d353" = 12
  dimension "d354" = 43.5
  dimension "d355" = 4
  dimension "d356" = 12
  dimension "d357" = 1
  dimension "d358" = 12
  dimension "d359" = 12
  dimension "d360" = 12
  dimension "d361" = 22.5
  dimension "d362" = 43.5
  dimension "d363" = 4
  dimension "d364" = 12
  dimension "d365" = 1
  dimension "d366" = 12
  dimension "d367" = 12
  dimension "d368" = 12
  dimension "d369" = 43.5
  dimension "d370" = 4
  dimension "d371" = 12
  dimension "d372" = 1
  dimension "d373" = 12
  dimension "d374" = 12
  dimension "d375" = 12
  dimension "d376" = 22.5
  dimension "d377" = 43.5
  dimension "d378" = 4
  dimension "d379" = 12
  dimension "d380" = 1
  dimension "d381" = 12
  dimension "d382" = 12
  dimension "d383" = 12
  dimension "d384" = 43.5
  dimension "d385" = 4
  dimension "d386" = 12
  dimension "d387" = 1
  dimension "d388" = 12
  dimension "d389" = 12
  dimension "d390" = 12
  dimension "d391" = 22.5
  constraint vertical L0
  constraint parallel L0 L2
  constraint horizontal L4
  constraint vertical L5
  constraint horizontal L6
  constraint vertical L7
  constraint vertical L9
  constraint horizontal L10
  constraint parallel L10 L11
  constraint horizontal L13
  constraint vertical L14
  constraint horizontal L15
  constraint vertical L24
  constraint coincident L12 L24.end
  constraint vertical L25
  constraint coincident L12 L25.end
  constraint midpoint L12 L28.start
  constraint coincident L12 L9.start
  constraint horizontal L29
  constraint vertical L30
  constraint horizontal L31
  constraint vertical L32
  constraint coincident P14 P12
  constraint coincident P13 P10
  constraint coincident P30 P28
  constraint coincident P27 P24
  constraint coincident P44 P42
  constraint coincident P43 P40
  constraint coincident P39 P38
  constraint coincident P62 P60
  constraint coincident P59 P56
  measures "d8" distance of L1.end L4.end
  measures "d26" distance of L10.end L11.start
  measures "d27" distance of L11.start L13.end
  measures "d132" distance of L17.end L19.start
  measures "d137" distance of L9.start L29.end
  measures "d138" distance of L9.start L31.end
  measures "d139" diameter of A0
  measures "d140" diameter of A1
  measures "d145" distance of L29 A0.centre
  measures "d146" distance of L31 A1.centre
  measures "d147" distance of L1 A0.centre
  measures "d148" distance of L0 A1.centre
  measures "d181" distance of L1.end L9.start
  measures "d182" distance of L4.end L5.end
  measures "d184" distance of L6.end L31.end
extrude "Extrusion1" add sketch "Skizze1" against normal blind 5 contours L0 L9 L10 L11 L12 L13 L14 L15 L22 L23 L24 L25 L26 L27 L29 L30 L31 | L0 L12 L28 L29 L30 L31 L32 | L0 L4 L5 L6 L12 L28 L32 | L16 L17 L18 L19 L20 L21 | A0 | A1 makes body 1 in component "Board"
extrude "Extrusion18" add sketch "Skizze1" along normal blind 5 contours L0 L12 L28 L29 L30 L31 L32 | L0 L4 L5 L6 L12 L28 L32 bodies 1 in component "Board"
extrude "Extrusion5" add sketch "Skizze1" along normal blind 40 separate body contours L16 L17 L18 L19 L20 L21 makes body 2 in component "Board"
sketch "Skizze3" plane through (0, 40, 0) normal (0, 1, 0) x (-1, 0, 0) in component "Board"
  line L0 (-99.5, -95.5) -> (-99.5, -42.25)
  line L1 (-99.5, -26.25) -> (-99.5, 28.5)
  line L2 (-99.5, 28.5) -> (50, 28.5)
  line L3 (50, 28.5) -> (50, -95.5)
  line L4 (50, -95.5) -> (-99.5, -95.5)
  line L5 (-104.5, -100.5) -> (55, -100.5)
  line L6 (55, -100.5) -> (55, 33.5)
  line L7 (55, 33.5) -> (-104.5, 33.5)
  line L8 (-104.5, 33.5) -> (-104.5, -100.5)
  line L9 (-99.5, -42.25) -> (-99.5, -25.5)
  line L10 (-104.5, 33.5) -> (-104.5, -100.5)
  line L11 (-104.5, -100.5) -> (55, -100.5)
  line L12 (55, 33.5) -> (0, 33.5)
  line L13 (55, -100.5) -> (55, 33.5)
  line L14 (0, -100.5) -> (55, -100.5)
  line L15 (0, -100.5) -> (-104.5, -100.5)
  line L16 (-104.5, 33.5) -> (0, 33.5)
  line L17 (-104.5, -100.5) -> (-104.5, 33.5)
  line L18 (-99.5, -95.5) -> (-99.5, 28.5)
  line L19 (0, -95.5) -> (50, -95.5)
  line L20 (50, 28.5) -> (0, 28.5)
  line L21 (50, -95.5) -> (50, 28.5)
  line L22 (0, -95.5) -> (-99.5, -95.5)
  line L23 (-99.5, 28.5) -> (0, 28.5)
sketch "Skizze4" plane through (-55, 0, 0) normal (-1, 0, 0) x (0, 0, 1) in component "Board"
  line L0 (-100.5, 0) -> (33.5, 0)
  line L1 (33.5, 0) -> (33.5, 40)
  line L2 (33.5, 40) -> (-100.5, 40)
  line L3 (-100.5, 40) -> (-100.5, 0)
  line L4 (-100.5, 40) -> (-93.5, 40)
  line L5 (-93.5, 40) -> (-93.5, 0)
  line L6 (-93.5, 0) -> (-100.5, 0)
  line L7 (-100.5, 0) -> (-100.5, 40)
  line L8 (-93.5, 40) -> (-63.5, 40)
  line L9 (-63.5, 40) -> (-63.5, 0)
  line L10 (-63.5, 0) -> (-93.5, 0)
  line L11 (-93.5, 0) -> (-93.5, 40)
  line L12 (-100.5, 20) -> (-93.5, 20) construction
  line L13 (-93.5, 20) -> (-63.5, 20) construction
  line L14 (-63.5, 20) -> (-33.5, 20) construction
  line L15 (-33.5, 20) -> (-3.5, 20) construction
  line L16 (-3.5, 20) -> (26.5, 20) construction
  circle A0 centre (-78.5, 17.6) radius 12
  line L17 (-65.4, 2.1) -> (-91.6, 2.1)
  line L18 (-91.6, 2.1) -> (-91.6, 33.1)
  line L19 (-91.6, 33.1) -> (-65.4, 33.1)
  line L20 (-65.4, 33.1) -> (-65.4, 2.1)
  line L21 (-65.4, 2.1) -> (-91.6, 33.1) construction
  line L22 (-91.6, 2.1) -> (-65.4, 33.1) construction
  line L23 (-91.6, 33.1) -> (-88.1, 33.1) construction
  line L24 (-88.1, 33.1) -> (-88.1, 29.6) construction
  line L25 (-88.1, 29.6) -> (-91.6, 29.6) construction
  line L26 (-91.6, 29.6) -> (-91.6, 33.1) construction
  line L27 (-65.4, 2.1) -> (-68.9, 2.1) construction
  line L28 (-68.9, 2.1) -> (-68.9, 5.6) construction
  line L29 (-68.9, 5.6) -> (-65.4, 5.6) construction
  line L30 (-65.4, 5.6) -> (-65.4, 2.1) construction
  circle A1 centre (-88.1, 29.6) radius 1.5
  circle A2 centre (-68.9, 5.6) radius 1.5
  line L31 (-61.6, 2.1) -> (-61.6, 33.1)
  line L32 (-61.6, 33.1) -> (-35.4, 33.1)
  line L33 (-35.4, 2.1) -> (-61.6, 2.1)
  line L34 (-35.4, 33.1) -> (-35.4, 2.1)
  circle A3 centre (-48.5, 17.6) radius 12
  circle A4 centre (-58.1, 29.6) radius 1.5
  circle A5 centre (-38.9, 5.6) radius 1.5
  line L35 (-31.6, 2.1) -> (-31.6, 33.1)
  line L36 (-31.6, 33.1) -> (-5.4, 33.1)
  line L37 (-5.4, 2.1) -> (-31.6, 2.1)
  line L38 (-5.4, 33.1) -> (-5.4, 2.1)
  circle A6 centre (-18.5, 17.6) radius 12
  circle A7 centre (-28.1, 29.6) radius 1.5
  circle A8 centre (-8.9, 5.6) radius 1.5
  line L39 (-1.6, 2.1) -> (-1.6, 33.1)
  line L40 (-1.6, 33.1) -> (24.6, 33.1)
  line L41 (24.6, 2.1) -> (-1.6, 2.1)
  line L42 (24.6, 33.1) -> (24.6, 2.1)
  circle A9 centre (11.5, 17.6) radius 12
  circle A10 centre (1.9, 29.6) radius 1.5
  circle A11 centre (21.1, 5.6) radius 1.5
  point P0 (-78.5, 17.6)
  dimension "d43" = 7
  dimension "d44" = 30
  dimension "d49" = 24
  dimension "d50" = 26.2
  dimension "d51" = 31
  dimension "d52" = 3.5
  dimension "d53" = 3.5
  dimension "d54" = 3.5
  dimension "d55" = 3.5
  dimension "d56" = 3
  dimension "d57" = 3
  dimension "d60" = 90
  dimension "d61" = 0
  constraint horizontal L4
  constraint vertical L5
  constraint horizontal L6
  constraint vertical L7
  constraint coincident L2.end L3.start
  constraint horizontal L8
  constraint vertical L9
  constraint horizontal L10
  constraint vertical L11
  constraint midpoint L7 L12.start
  constraint midpoint L11 L12.end
  constraint perpendicular L11 L12
  constraint horizontal L17
  constraint perpendicular L17 L18
  constraint parallel L17 L19
  constraint parallel L18 L20
  constraint coincident L21 P0
  constraint coincident L22 P0
  constraint coincident P0 A0.centre
  constraint horizontal L23
  constraint vertical L24
  constraint horizontal L25
  constraint vertical L26
  constraint horizontal L27
  constraint vertical L28
  constraint horizontal L29
  constraint vertical L30
  constraint coincident L24.end L25.start
  constraint coincident L28.end L29.start
  measures "d43" distance of L2.end L4.end
  measures "d44" distance of L4.end L8.end
  measures "d49" diameter of A0
  measures "d50" distance of L18.end L19.end
  measures "d51" distance of L17.end L18.end
  measures "d52" distance of L18.end L23.end
  measures "d53" distance of L18.end L25.end
  measures "d54" distance of L17.start L27.end
  measures "d55" distance of L17.start L29.end
  measures "d56" diameter of A1
  measures "d57" diameter of A2
extrude "Extrusion6" add sketch "Skizze3" along normal blind 5 separate body contours L0 L1 L2 L3 L4 L9 L18 L19 L20 L21 L22 L23 | L5 L6 L7 L8 L10 L11 L12 L13 L14 L15 L16 L17 makes body 3 in component "Board"
extrude "Extrusion7" cut sketch "Skizze4" against normal up to surface (5 mm away) contours A0 | A1 | A2 | A3 | A4 | A5 | A6 | A7 | A8 | A9 | A10 | A11 bodies 2 in component "Board"
extrude "Extrusion8" add 1 faces at (-50, 37.0329, -31.6788) along direction (1, 0, 0) blind 5 on bodies 2 bodies 2 1 in component "Board"
sketch "Skizze5" plane through (0, 40, 0) normal (0, -1, 0) x (1, 0, 0) in component "Board"
  line L0 (-55, -100.5) -> (104.5, -100.5)
  line L1 (104.5, -100.5) -> (104.5, 33.5)
  line L2 (104.5, 33.5) -> (-55, 33.5)
  line L3 (-55, 33.5) -> (-55, -100.5)
  line L4 (-50, 28.5) -> (0, 28.5)
  line L5 (99.5, -95.5) -> (99.5, 28.5)
  line L6 (0, -95.5) -> (99.5, -95.5)
  line L7 (0, -95.5) -> (-50, -95.5)
  line L8 (-50, -95.5) -> (-50, 28.5)
  line L9 (99.5, 28.5) -> (0, 28.5)
  line L10 (-55, 33.5) -> (0, 33.5)
  line L11 (-55, -100.5) -> (-55, 33.5)
  line L12 (104.5, 33.5) -> (0, 33.5)
  line L13 (104.5, -100.5) -> (104.5, 33.5)
  line L14 (0, -100.5) -> (104.5, -100.5)
  line L15 (-50, 28.5) -> (-40, 28.5)
  line L16 (-40, 28.5) -> (-40, 18.5)
  line L17 (-40, 18.5) -> (-50, 18.5)
  line L18 (-50, 18.5) -> (-50, 28.5)
  line L19 (99.5, 28.5) -> (89.5, 28.5)
  line L20 (89.5, 28.5) -> (89.5, 18.5)
  line L21 (89.5, 18.5) -> (99.5, 18.5)
  line L22 (99.5, 18.5) -> (99.5, 28.5)
  line L23 (99.5, -95.5) -> (89.5, -95.5)
  line L24 (89.5, -95.5) -> (89.5, -85.5)
  line L25 (89.5, -85.5) -> (99.5, -85.5)
  line L26 (99.5, -85.5) -> (99.5, -95.5)
  line L27 (-50, -95.5) -> (-40, -95.5)
  line L28 (-40, -95.5) -> (-40, -85.5)
  line L29 (-40, -85.5) -> (-50, -85.5)
  line L30 (-50, -85.5) -> (-50, -95.5)
  line L31 (-50, 23.5) -> (-40, 23.5) construction
  line L32 (89.5, 23.5) -> (99.5, 23.5) construction
  line L33 (94.5, 28.5) -> (94.5, 18.5) construction
  line L34 (94.5, -85.5) -> (94.5, -95.5) construction
  line L35 (99.5, -90.5) -> (89.5, -90.5) construction
  line L36 (-40, -90.5) -> (-50, -90.5) construction
  line L37 (-45, -95.5) -> (-45, -85.5) construction
  line L38 (-45, 18.5) -> (-45, 28.5) construction
  circle A0 centre (-45, 23.5) radius 1.5
  circle A1 centre (94.5, 23.5) radius 1.5
  circle A2 centre (94.5, -90.5) radius 1.5
  circle A3 centre (-45, -90.5) radius 1.5
  dimension "d66" = 10
  dimension "d67" = 10
  dimension "d68" = 10
  dimension "d69" = 10
  dimension "d70" = 10
  dimension "d71" = 10
  dimension "d72" = 10
  dimension "d73" = 10
  dimension "d74" = 3
  dimension "d75" = 3
  dimension "d76" = 3
  dimension "d77" = 3
  constraint horizontal L15
  constraint vertical L16
  constraint horizontal L17
  constraint vertical L18
  constraint coincident L4.start L8.end
  constraint horizontal L19
  constraint vertical L20
  constraint horizontal L21
  constraint vertical L22
  constraint coincident L5.end L9.start
  constraint horizontal L23
  constraint vertical L24
  constraint horizontal L25
  constraint vertical L26
  constraint coincident L5.start L6.end
  constraint horizontal L27
  constraint vertical L28
  constraint horizontal L29
  constraint vertical L30
  constraint coincident L7.end L8.start
  constraint midpoint L18 L31.start
  constraint midpoint L16 L31.end
  constraint midpoint L20 L32.start
  constraint midpoint L22 L32.end
  constraint midpoint L19 L33.start
  constraint midpoint L21 L33.end
  constraint midpoint L25 L34.start
  constraint midpoint L23 L34.end
  constraint midpoint L26 L35.start
  constraint midpoint L24 L35.end
  constraint midpoint L28 L36.start
  constraint midpoint L30 L36.end
  constraint midpoint L27 L37.start
  constraint midpoint L29 L37.end
  constraint midpoint L17 L38.start
  constraint midpoint L15 L38.end
  constraint midpoint L38 A0.centre
  constraint midpoint L32 A1.centre
  constraint midpoint L35 A2.centre
  constraint midpoint L37 A3.centre
  measures "d66" distance of L4.start L15.end
  measures "d67" distance of L4.start L17.end
  measures "d68" distance of L5.end L19.end
  measures "d69" distance of L5.end L21.end
  measures "d70" distance of L5.start L23.end
  measures "d71" distance of L5.start L25.end
  measures "d72" distance of L7.end L27.end
  measures "d73" distance of L7.end L29.end
  measures "d74" diameter of A0
  measures "d75" diameter of A1
  measures "d76" diameter of A2
  measures "d77" diameter of A3
extrude "Extrusion9" cut sketch "Skizze5" against normal up to surface (5 mm away) contours A0 | A1 | A2 | A3 bodies 3 in component "Board"
extrude "Extrusion10" add sketch "Skizze5" along normal blind 20 separate body contours L4 L8 L15 L16 L17 L18 | L7 L8 L27 L28 L29 L30 | L5 L9 L19 L20 L21 L22 | L5 L6 L23 L24 L25 L26 makes body 4 at (-46.6667, 33.3333, 28.5) makes body 5 at (-43.3333, 33.3333, -85.5) makes body 6 at (99.5, 26.6667, 21.8333) makes body 7 at (99.5, 33.3333, -92.1667) in component "Board"
chamfer "Fase1" distance 10 angle 45 4 edges at (-45, 20, 18.5) (94.5, 20, -85.5) (94.5, 20, 18.5) (-45, 20, -85.5) on bodies 4 5 6 7 in component "Board"
extrude "Extrusion11" cut sketch "Skizze5" along normal blind 14 contours A0 | A3 bodies 2 in component "Board"